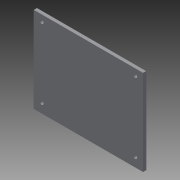
# Autodesk Inventor part: top panel
Saved by Autodesk Inventor 2014 (Build 180170000, 170)
## iProperties
Created: 2014-11-30
Part Number: top panel
Material: Generic
Document SubType Name: Modeling
Designer: ph1140784
Density: 1 g/cm^3
Appearance: Default
Author: ph1140784
Autodesk Inventor part; units mm, degrees
ref_plane "YZ Plane" through (0, 0, 0) normal (1, 0, 0) x (0, 1, 0)
ref_plane "XZ Plane" through (0, 0, 0) normal (0, 1, 0) x (-1, 0, 0)
ref_plane "XY Plane" through (0, 0, 0) normal (0, 0, 1) x (1, 0, 0)
ref_plane "Work Plane1" through (0, 3, 0) normal (0, 1, 0) x (1, 0, 0)
sketch "Sketch2" plane through (0, 3, 0) normal (0, 1, 0) x (1, 0, 0)
  line L0 (0, 0) -> (0, 20)
  line L1 (20, 0) -> (0, 0)
  line L2 (0, 0) -> (140, 0)
  line L3 (140, 0) -> (140, 110)
  line L4 (0, 110) -> (0, 0)
  line L5 (0, 110) -> (140, 110)
  circle A0 centre (10, 98) radius 2.5
  circle A1 centre (10, 8) radius 2.5
  circle A2 centre (130, 98) radius 2.5
  circle A3 centre (130, 8) radius 2.5
  constraints: 12 end point, 4 centre point, 2 perpendicular, 1 horizontal, 1 parallel
extrude "Extrusion3" add sketch "Sketch2" along normal blind 4
body "Solid3"
